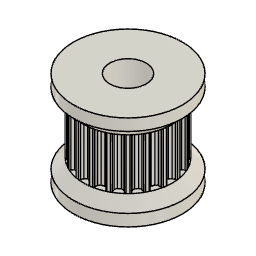
Parametric GT2 Pulley v9 (Autodesk Fusion 360 design; units mm, degrees)
Autodesk Fusion 360 part; units mm, degrees
sketch "Footprint" plane through (0, 0, 0) normal (0, 0, 1) x (1, 0, 0) in component "GT2 Pulley"
  circle A0 centre (0, 0) radius 7.5
  circle A1 centre (0, 0) radius 2.5
  dimension "d9" = 5
  dimension "d10" = 15
  constraint coincident A0.centre A1.centre
  measures "d9" diameter of A1
  measures "d10" diameter of A0
sketch "GT2 Profile" plane through (0, 0, 0) normal (0, 0, 1) x (1, 0, 0) in component "GT2 Pulley"
  circle A0 centre (0, 0) radius 6.3662 construction
  circle A1 centre (0, 0) radius 6.1122
  circle A2 centre (0, 0) radius 5.3622
  line L0 (0, 0) -> (0, 6.3662) construction
  line L1 (0, 0) -> (0.3997, 6.3536) construction
  line L2 (0, 0) -> (-0.3997, 6.3536) construction
  arc A3 (-0.616, 6.0811) -> (-0.4801, 5.5965) centre (0.3838, 6.1001) ccw
  arc A4 (0.4787, 5.594) -> (0.616, 6.0811) centre (-0.3838, 6.1001) ccw
  arc A5 (-0.5113, 6.0908) -> (0.5113, 6.0908) centre (0, 5.8749) ccw
  circle A6 centre (-0.7512, 5.9147) radius 0.15
  circle A7 centre (0.7512, 5.9147) radius 0.15
  dimension "d12" = 12.7324
  dimension "d24" = 3.6
  dimension "d25" = 3.6
  dimension "d28" = 1
  dimension "d29" = 0.555
  dimension "d30" = 1
  dimension "d32" = 0.15
  dimension "d33" = 0.15
  dimension "d45" = 12.2244
  dimension "d46" = 10.7244
  constraint coincident A0.centre A1.centre
  constraint coincident A0 L0.end
  constraint vertical L0
  constraint coincident L0 A5.centre
  constraint coincident A0 L1.end
  constraint coincident A0 L2.end
  constraint coincident A1 A3.centre
  constraint coincident L1 A3.centre
  constraint coincident A1 A4.centre
  constraint coincident L2 A4.centre
  constraint coincident A1 A3.start
  constraint coincident A1 A4.end
  constraint coincident A1 A5.end
  constraint coincident A1 A5.start
  constraint tangent A1 A6
  constraint tangent A3 A6
  constraint tangent A4 A5
  constraint tangent A4 A7
  constraint tangent A1 A7
  constraint coincident A5 A3.end
  constraint coincident A5 A4.start
  measures "d12" diameter of A0
  measures "d24" angle of L0 L1
  measures "d25" angle of L0 L2
  measures "d28" radius of A4
  measures "d29" radius of A5
  measures "d30" radius of A3
  measures "d32" radius of A6
  measures "d33" radius of A7
  measures "d45" diameter of A1
  measures "d46" diameter of A2
extrude "Extrude1" add sketch "Footprint" along normal blind 3 contours A0 | A1 in component "GT2 Pulley"
extrude "Extrude2" add sketch "GT2 Profile" along normal blind 7 from surface at 3 in component "GT2 Pulley"
extrude "Extrude3" add sketch "Footprint" along normal blind 3 from surface at 10 contours A0 | A1 in component "GT2 Pulley"
chamfer "Chamfer1" distance 1.3878 angle 45 2 edges at (-6.9925, -2.7121, 10) (-6.9925, -2.7121, 3) in component "GT2 Pulley"
extrude "Extrude5" cut sketch "GT2 Profile" along normal blind 7 from surface at 3 contours A1 A4 A5 | A1 A4 A7 | A1 A2 A5 | A1 A3 A5 | A1 A3 A6 in component "GT2 Pulley"
pattern_circular "C-Pattern2" count 20 over 360 about axis through (0, 0, 1.75) along (0, 0, 1) of "Extrude5" in component "GT2 Pulley"
extrude "Extrude4" cut sketch "Footprint" along normal through all contours A1 in component "GT2 Pulley"
component "GT2 Pulley" placed x (1, 0, 0) y (0, 1, 0) z (0, 0, 1) at (0, 0, 0)
equation "GT2_PULLEY_XY_OUTER_DIAMETER = 15 mm"
equation "GT2_PULLEY_Z_FACE_WIDTH = 7 mm"
equation "GT2_PULLEY_Z_LIP_THICKNESS = 3 mm"
equation "GT2_PULLEY_PITCH = 2 mm"
equation "GT2_PULLEY_TEETH = 20"
equation "GT2_PULLEY_XY_BORE_DIAMETER = 5 mm"
equation "d9 = GT2_PULLEY_XY_BORE_DIAMETER"
equation "d10 = GT2_PULLEY_XY_OUTER_DIAMETER"
equation "d12 = GT2_PULLEY_XY_PITCH_DIAMETER"
equation "GT2_PULLEY_XY_PLD = 0.254 mm"
equation "GT2_PULLEY_XY_TIP_HEIGHT = 0.75 mm"
equation "d24 = ( ( 0.40 mm ) / ( GT2_PULLEY_PITCH * GT2_PULLEY_TEETH ) ) * 360 deg"
equation "d25 = ( ( 0.40 mm ) / ( GT2_PULLEY_PITCH * GT2_PULLEY_TEETH ) ) * 360 deg"
equation "d34 = GT2_PULLEY_Z_LIP_THICKNESS"
equation "d36 = GT2_PULLEY_Z_LIP_THICKNESS"
equation "d37 = GT2_PULLEY_Z_FACE_WIDTH"
equation "d39 = GT2_PULLEY_Z_LIP_THICKNESS + GT2_PULLEY_Z_FACE_WIDTH"
equation "d40 = GT2_PULLEY_Z_LIP_THICKNESS"
equation "GT2_PULLEY_XY_PITCH_DIAMETER = ( GT2_PULLEY_PITCH * GT2_PULLEY_TEETH ) / 3.14159"
equation "GT2_PULLEY_XY_TIP_DIAMETER = GT2_PULLEY_XY_PITCH_DIAMETER - ( 0.254 * 2 ) * 1 mm"
equation "GT2_PULLEY_XY_ROOT_DIAMETER = GT2_PULLEY_XY_TIP_DIAMETER - ( 0.75 * 2 ) * 1 mm"
equation "d45 = GT2_PULLEY_XY_TIP_DIAMETER"
equation "d46 = GT2_PULLEY_XY_ROOT_DIAMETER"
equation "d47 = ( GT2_PULLEY_XY_OUTER_DIAMETER - GT2_PULLEY_XY_TIP_DIAMETER ) / 2"
equation "d49 = GT2_PULLEY_Z_LIP_THICKNESS"
equation "d50 = GT2_PULLEY_Z_FACE_WIDTH"
equation "d54 = GT2_PULLEY_TEETH"
named bodies: "GT2 Pulley"
